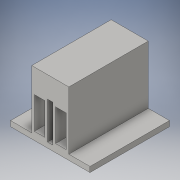
# Autodesk Inventor part: SupportForMotorMountV02
Saved by Autodesk Inventor 2016 SP1 (Build 200210100, 210)
## iProperties
Created: 2016-02-13
Part Number: SupportForMotorMountV02
Material: Generic
Document SubType Name: Modeling
Designer: steele
Density: 1 g/cm^3
Appearance: Default
Author: steele
Autodesk Inventor part; units mm, degrees
ref_plane "YZ Plane" through (0, 0, 0) normal (1, 0, 0) x (0, 1, 0)
ref_plane "XZ Plane" through (0, 0, 0) normal (0, 1, 0) x (-1, 0, 0)
ref_plane "XY Plane" through (0, 0, 0) normal (0, 0, 1) x (1, 0, 0)
sketch "Sketch1" plane through (0, 0, 0) normal (0, 1, 0) x (-1, 0, 0)
  line L0 (47.625, 47.625) -> (-47.625, 47.625)
  line L1 (-47.625, 47.625) -> (-47.625, -47.625)
  line L2 (-47.625, -47.625) -> (47.625, -47.625)
  line L3 (47.625, -47.625) -> (47.625, 47.625)
  line L4 (47.625, 47.625) -> (-47.625, -47.625) construction
  line L5 (-47.625, 47.625) -> (47.625, -47.625) construction
  point P0 (0, 0)
  dimension "d0" = 95.25
  dimension "d1" = 95.25
  constraints: 12 end point, 2 midpoint, 2 parallel, 1 horizontal, 1 perpendicular
  measures "d0" distance of L0.start L0.end
  measures "d1" distance of L2.end L0.start
extrude "Extrusion1" add sketch "Sketch1" along normal blind 6.35
sketch "Sketch2" plane through (-47.625, 0, 47.625) normal (0, 0, 1) x (1, 0, 0)
  line L0 (0, 6.35) -> (95.25, 6.35) projected
  line L1 (25.4, 6.35) -> (44.45, 6.35)
  line L2 (44.45, 6.35) -> (44.45, 50.8)
  line L3 (44.45, 50.8) -> (25.4, 50.8)
  line L4 (25.4, 50.8) -> (25.4, 6.35)
  line L5 (50.8, 6.35) -> (69.85, 6.35)
  line L6 (69.85, 6.35) -> (69.85, 50.8)
  line L7 (69.85, 50.8) -> (50.8, 50.8)
  line L8 (50.8, 50.8) -> (50.8, 6.35)
  line L9 (0, 0) -> (0, 6.35) projected
  line L10 (28.575, 9.525) -> (41.275, 9.525)
  line L11 (41.275, 9.525) -> (41.275, 47.625)
  line L12 (41.275, 47.625) -> (28.575, 47.625)
  line L13 (28.575, 47.625) -> (28.575, 9.525)
  line L14 (28.575, 9.525) -> (41.275, 47.625) construction
  line L15 (41.275, 9.525) -> (28.575, 47.625) construction
  line L16 (53.975, 9.525) -> (66.675, 9.525)
  line L17 (66.675, 9.525) -> (66.675, 47.625)
  line L18 (66.675, 47.625) -> (53.975, 47.625)
  line L19 (53.975, 47.625) -> (53.975, 9.525)
  line L20 (53.975, 9.525) -> (66.675, 47.625) construction
  line L21 (66.675, 9.525) -> (53.975, 47.625) construction
  point P0 (47.625, 0)
  point P1 (34.925, 28.575)
  point P2 (60.325, 28.575)
  dimension "d4" = 19.05
  dimension "d5" = 44.45
  dimension "d6" = 6.35
  dimension "d7" = 25.4
  dimension "d8" = 3.175
  dimension "d9" = 3.175
  dimension "d10" = 3.175
  dimension "d11" = 3.175
  dimension "d12" = 3.175
  dimension "d13" = 3.175
  constraints: 40 end point, 8 parallel, 5 perpendicular, 4 midpoint, 3 collinear, 3 horizontal, 3 point on line
  measures "d4" distance of L2.end L3.end
  measures "d5" distance of L3.end L1.start
  measures "d6" distance between parallel lines of L2 L8
  measures "d7" distance between parallel lines of L9 L4
  measures "d8" distance between parallel lines of L10 L0
  measures "d9" distance between parallel lines of L2 L11
  measures "d10" distance between parallel lines of L6 L17
  measures "d11" distance between parallel lines of L4 L13
  measures "d12" distance between parallel lines of L19 L8
  measures "d13" distance between parallel lines of L3 L12
extrude "Extrusion2" add sketch "Sketch2" against normal blind 95.25
sketch "Sketch3" plane through (-22.225, 50.8, 47.625) normal (0, 1, 0) x (1, 0, 0)
  line L0 (0, 0) -> (0, 95.25) projected
  line L1 (0, 0) -> (44.45, 0)
  line L2 (44.45, 0) -> (44.45, 95.25)
  line L3 (44.45, 95.25) -> (0, 95.25)
  line L4 (0, 95.25) -> (0, 0)
  point P0 (22.225, 47.625)
  constraints: 8 end point, 2 parallel, 1 horizontal, 1 perpendicular
extrude "Extrusion3" add sketch "Sketch3" along normal blind 25.4
equation "\"d0\" = width"
equation "\"d1\" = length"
equation "\"d2\" = thickness"
equation "\"d4\" = tubeWidth"
equation "\"d5\" = tubeLength"
equation "\"d8\" = tubeWallThickness"
equation "\"d9\" = tubeWallThickness"
equation "\"d10\" = tubeWallThickness"
equation "\"d11\" = tubeWallThickness"
equation "\"d12\" = tubeWallThickness"
equation "\"d13\" = tubeWallThickness"
equation "\"d14\" = length"
equation "\"length\" = 95.25"
equation "\"width\" = 95.25"
equation "\"thickness\" = 6.35"
equation "\"tubeLength\" = 44.45"
equation "\"tubeWidth\" = 19.05"
equation "\"tubeWallThickness\" = 3.175"
body "Solid1"
